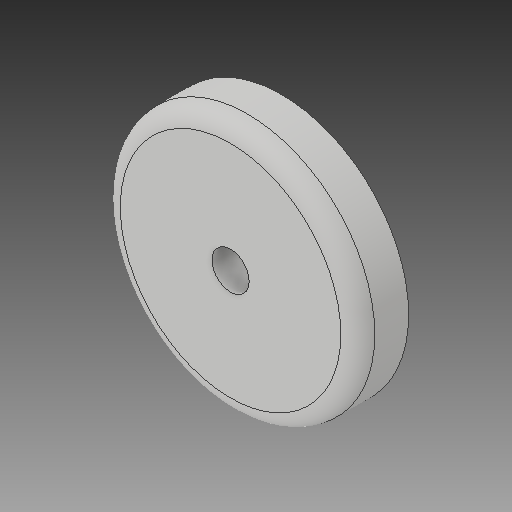
# Autodesk Inventor part: крышка
Saved by Autodesk Inventor 2019 (Build 230136000, 136)
## iProperties
Created: 2018-01-17
Part Number: крышка
Material: Типовые
Document SubType Name: Modeling
Designer: olege
Density: 1 g/cm^3
Appearance: По умолчанию
Mass: 1.8297 g
Surface Area: 16.4157 cm^2
Volume: 1.8297 cm^3
Author: olege
Autodesk Inventor part; units mm, degrees
ref_plane "YZ Plane" through (0, 0, 0) normal (1, 0, 0) x (0, 1, 0)
ref_plane "XZ Plane" through (0, 0, 0) normal (0, 1, 0) x (-1, 0, 0)
ref_plane "XY Plane" through (0, 0, 0) normal (0, 0, 1) x (1, 0, 0)
sketch "Эскиз1" plane through (0, 0, 0) normal (0, 0, 1) x (1, 0, 0)
  circle A0 centre (0, 0) radius 15
  circle A1 centre (0, 6.5) radius 1.35 construction
  circle A2 centre (-5.6292, -3.25) radius 1.35 construction
  circle A3 centre (5.6292, -3.25) radius 1.35 construction
  circle A4 centre (0, 0) radius 1.1
  dimension "d0" = 30
  dimension "d1" = 2.7
  dimension "d2" = 6.5
  dimension "d5" = 360
  dimension "d21" = 2.2
  constraints: 5 centre point, 2 coincident, 1 vertical alignment, 7 other
  measures "d0" diameter of A0
  measures "d1" diameter of A1
  measures "d2" distance of point (0, 0) A1.centre
  measures "d21" diameter of A4
extrude "Выдавливание1" add sketch "Эскиз1" along normal blind 6 contours A0 | A4
fillet "Сопряжение1" radius 2 1 edges at (-15, 0, 6)
sketch "Эскиз4" plane through (0, 0, 6) normal (0, 0, 1) x (1, 0, 0)
  circle A0 centre (0, 0) radius 2.2
  dimension "d22" = 4.4
  constraints: 1 centre point, 1 coincident
  measures "d22" diameter of A0
extrude "Выдавливание4" cut sketch "Эскиз4" against normal blind 10
sketch "Эскиз5" plane through (0, 0, 0) normal (0, 0, -1) x (-1, 0, 0)
  circle A0 centre (0, 0) radius 9.15
  dimension "d28" = 18.3
  constraints: 1 centre point, 1 coincident
  measures "d28" diameter of A0
extrude "Выдавливание5" cut sketch "Эскиз5" against normal blind 0.8
